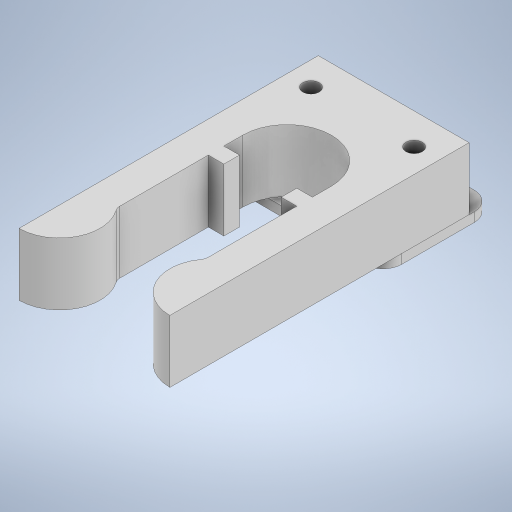
# Autodesk Inventor part: Clip brazo
Saved by Autodesk Inventor 2023 (Build 270158000, 158)
## iProperties
Created: 2022-05-26
Part Number: Clip brazo
Material: Generic
Document SubType Name: Modeling
Designer: juanp
Density: 1 g/cm^3
Appearance: Default
Author: juanp
Autodesk Inventor part; units mm, degrees
ref_plane "YZ Plane" through (0, 0, 0) normal (1, 0, 0) x (0, 1, 0)
ref_plane "XZ Plane" through (0, 0, 0) normal (0, 1, 0) x (-1, 0, 0)
ref_plane "XY Plane" through (0, 0, 0) normal (0, 0, 1) x (1, 0, 0)
sketch "Sketch1" plane through (0, 0, 0) normal (0, 1, 0) x (-1, 0, 0)
  line L0 (14.2, 73.7) -> (-14.2, 73.7) construction
  line L1 (-14.2, 73.7) -> (-14.2, 20)
  line L2 (-14.2, 20) -> (14.2, 20) construction
  line L3 (14.2, 20) -> (14.2, 73.7)
  line L4 (-24.2, 96.0274) -> (-24.2, 20)
  line L5 (24.2, 96.0274) -> (24.2, 20)
  line L6 (-24.2, 20) -> (-14.2, 20)
  line L7 (24.2, 20) -> (14.2, 20)
  line L8 (-24.2, 0) -> (24.2, 0)
  line L9 (24.2, 0) -> (24.2, 20)
  line L10 (24.2, 20) -> (-24.2, 20)
  line L11 (-24.2, 20) -> (-24.2, 0)
  arc A0 (-13.6375, 75.4489) -> (-14.2, 73.7) centre (-11.2, 73.7) ccw
  arc A1 (14.2, 73.7) -> (13.6375, 75.4489) centre (11.2, 73.7) ccw
  arc A2 (24.2, 96.0274) -> (13.6375, 75.4489) centre (24.2, 83.0274) ccw
  arc A3 (-13.6375, 75.4489) -> (-24.2, 96.0274) centre (-24.2, 83.0274) ccw
  line L12 (11.2, 89.334) -> (11.2, 76.7208) construction
  line L13 (-11.2, 89.334) -> (-11.2, 76.7208) construction
  line L14 (-14.2, 73.7) -> (14.2, 73.7)
  line L15 (14.2, 73.7) -> (14.2, 45.3)
  line L16 (14.2, 45.3) -> (-14.2, 45.3)
  line L17 (-14.2, 45.3) -> (-14.2, 73.7)
  line L18 (-14.2, 45.3) -> (-9.2, 45.3)
  line L19 (-9.2, 45.3) -> (-9.2, 40.3)
  line L20 (-9.2, 40.3) -> (-14.2, 40.3)
  line L21 (-14.2, 40.3) -> (-14.2, 45.3)
  line L22 (14.2, 45.3) -> (9.2, 45.3)
  line L23 (9.2, 45.3) -> (9.2, 40.3)
  line L24 (9.2, 40.3) -> (14.2, 40.3)
  line L25 (14.2, 40.3) -> (14.2, 45.3)
  point P0 (0, 0)
  point P1 (0, 0)
  point P2 (-11.2, 83.0274)
  point P3 (11.2, 83.0274)
  point P4 (-11.7, 45.3)
  point P5 (-11.7, 40.3)
  dimension "d0" = 28.4
  dimension "d2" = 3
  dimension "d4" = 3
  dimension "d5" = 3
  dimension "d6" = 20
  dimension "d7" = 10
  dimension "d13" = 53.7
  dimension "d40" = 5
  dimension "d41" = 5
  constraints: 52 end point, 16 equal length, 10 point on circle, 6 horizontal, 6 tangent, 5 midpoint, 5 perpendicular, 4 centre point, 4 vertical, 2 equal radius, 1 coincident, 1 line through centre, 1 point on line, 1 other
  measures "d0" distance of L0.start L0.end
  measures "d2" radius of A0
  measures "d4" distance between parallel lines of L12 L3
  measures "d5" distance between parallel lines of L1 L13
  measures "d6" distance between parallel lines of L8 L10
  measures "d7" distance between parallel lines of L4 L1
  measures "d13" distance of L0.end L1.end
  measures "d40" distance of L23.end L24.end
  measures "d41" distance of point (-11.7, 45.3) point (-11.7, 40.3)
extrude "Extrusion1" add sketch "Sketch1" along normal blind 20 contours L1 L6 L4 A3 A0 | L16 L19 L20 L1 | A1 A2 L5 L7 L3 | L3 L24 L23 L16 | L10 L7 L9 L8 L11 L6
sketch "Sketch2" plane through (0, 20, 0) normal (0, 1, 0) x (1, 0, 0)
  line L0 (-14.2, -20) -> (14.2, -20) projected
  line L1 (0, -20) -> (0, 0) construction
  line L2 (24.2, -96.0274) -> (24.2, 0) projected
  line L3 (-24.2, 0) -> (-24.2, -96.0274) projected
  circle A0 centre (-16.55, -10) radius 2.65
  circle A1 centre (16.55, -10) radius 2.65
  line L4 (0, -10) -> (-24.2, -10) construction
  line L5 (-24.2, 0) -> (-24.2, -96.0274) projected
  line L6 (0, -10) -> (24.2, -10) construction
  dimension "d10" = 5.3
  dimension "d28" = 5
  dimension "d29" = 5
  constraints: 6 end point, 5 point on line, 2 centre point, 2 midpoint, 1 equal radius, 1 perpendicular, 1 vertical
  measures "d10" diameter of A1
  measures "d28" distance edge to line of A0 L3
  measures "d29" distance edge to line of A1 L2
extrude "Extrusion2" cut sketch "Sketch2" against normal through all
fillet "Fillet1" radius 14.2 2 edges at (-14.2, 10, 20) (14.2, 10, 20)
sketch "Sketch4" plane through (0, 0, 0) normal (0, 1, 0) x (1, 0, 0)
  line L0 (-16.55, 0) -> (-16.55, -20) construction
  line L1 (-19.2, 0) -> (-19.2, -20)
  line L2 (-13.9, -20) -> (-13.9, 0)
  arc A0 (-13.9, 0) -> (-19.2, 0) centre (-16.55, 0) ccw
  arc A1 (-19.2, -20) -> (-13.9, -20) centre (-16.55, -20) ccw
  line L3 (16.55, 0) -> (16.55, -20) construction
  line L4 (13.9, 0) -> (13.9, -20)
  line L5 (19.2, -20) -> (19.2, 0)
  arc A2 (19.2, 0) -> (13.9, 0) centre (16.55, 0) ccw
  arc A3 (13.9, -20) -> (19.2, -20) centre (16.55, -20) ccw
  circle A4 centre (-16.55, -10) radius 2.65 projected
  circle A5 centre (16.55, -10) radius 2.65 projected
  circle A6 centre (16.55, -10) radius 2.65 projected
  circle A7 centre (-16.55, -10) radius 2.65 projected
  line L6 (-14.2, -73.7) -> (-14.2, -45.3) projected
  arc A8 (14.2, -34.2) -> (-14.2, -34.2) centre (0, -34.2) ccw projected
  line L7 (14.2, -34.2) -> (14.2, -40.3) projected
  arc A9 (13.6375, -75.4489) -> (14.2, -73.7) centre (11.2, -73.7) ccw projected
  arc A10 (13.6375, -75.4489) -> (24.2, -96.0274) centre (24.2, -83.0274) ccw projected
  line L8 (24.2, -96.0274) -> (24.2, 0) projected
  line L9 (24.2, 0) -> (-24.2, 0) projected
  line L10 (-24.2, 0) -> (-24.2, -96.0274) projected
  arc A11 (-24.2, -96.0274) -> (-13.6375, -75.4489) centre (-24.2, -83.0274) ccw projected
  arc A12 (-14.2, -73.7) -> (-13.6375, -75.4489) centre (-11.2, -73.7) ccw projected
  line L11 (-24.2, -27.65) -> (24.2, -27.65)
  line L12 (24.2, -27.65) -> (24.2, 7.65)
  line L13 (24.2, 7.65) -> (-24.2, 7.65)
  line L14 (-24.2, 7.65) -> (-24.2, -27.65)
  line L15 (-14.2, -45.3) -> (-9.2, -45.3) projected
  line L16 (-9.2, -45.3) -> (-9.2, -40.3) projected
  line L17 (-9.2, -40.3) -> (-14.2, -40.3) projected
  line L18 (-14.2, -40.3) -> (-14.2, -34.2) projected
  line L19 (14.2, -40.3) -> (9.2, -40.3) projected
  line L20 (9.2, -40.3) -> (9.2, -45.3) projected
  line L21 (9.2, -45.3) -> (14.2, -45.3) projected
  line L22 (14.2, -45.3) -> (14.2, -73.7) projected
  point P0 (0, 0)
  point P1 (-16.55, 2.65)
  point P2 (-16.55, -22.65)
  point P3 (-24.2, 0)
  dimension "d15" = 20
  dimension "d16" = 5
  dimension "d17" = 5
  constraints: 24 end point, 10 point on circle, 8 tangent, 6 parallel, 4 centre point, 2 coincident, 2 equal radius, 2 midpoint, 2 point on line, 1 horizontal, 1 perpendicular, 1 vertical
  measures "d15" distance of L0.start L0.end
  measures "d16" distance from line of point (-16.55, 2.65) L13
  measures "d17" distance from line of point (-16.55, -22.65) L11
extrude "Extrusion3" add sketch "Sketch4" against normal blind 3 separate body contours L9 L14 L13 L12 A2 A0 | L1 A1 L2 L9 L4 A3 L5 L8 L11 A8 L10 | A8 L11
sketch "Sketch5" plane through (0, -3, 0) normal (0, -1, 0) x (1, 0, 0)
  line L0 (24.2, 27.65) -> (-24.2, 27.65) projected
  line L1 (0, 27.65) -> (0, -7.65)
  line L2 (-24.2, -7.65) -> (24.2, -7.65) projected
  line L3 (-3, 27.65) -> (-6, 27.65)
  line L4 (-6, 27.65) -> (-6, 18.05)
  line L5 (-6, 18.05) -> (-3, 18.05)
  line L6 (-3, 18.05) -> (-3, 27.65)
  point P0 (0, 0)
  point P1 (-4.5, 27.65)
  point P2 (-4.5, 18.05)
  point P3 (-6, 27.65)
  dimension "d20" = 3
  dimension "d21" = 3
  dimension "d37" = 9.6
  constraints: 10 end point, 4 midpoint, 2 parallel, 1 horizontal, 1 perpendicular, 1 point on line
  measures "d20" distance between parallel lines of L6 L1
  measures "d21" distance between parallel lines of L4 L6
  measures "d37" distance between parallel lines of L0 L5
extrude "Extrusion4" add sketch "Sketch5" along normal blind 20 bodies 2
chamfer "Chamfer1" distance 20 angle 45 1 edges at (-4.5, -3, 18.05)
fillet "Fillet2" radius 6 4 edges at (24.2, -1.5, 27.65) (24.2, -1.5, -7.65) (-24.2, -1.5, 27.65) (-24.2, -1.5, -7.65)
sketch "Sketch6" plane through (-3, -3, 27.65) normal (1, 0, 0) x (0, 0, -1)
  circle A0 centre (7.5, -15) radius 1
  circle A1 centre (7.5, -5) radius 1
  line L0 (7.5, -15) -> (7.5, -5) construction
  line L1 (0, 0) -> (0, -20) projected
  line L2 (6, 0) -> (0, 0) projected
  point P0 (27.65, 3)
  point P1 (0, -10)
  dimension "d33" = 10
  dimension "d34" = 2
  dimension "d38" = 7.5
  dimension "d39" = 5
  constraints: 2 centre point, 2 end point, 1 equal radius, 1 midpoint, 1 vertical
  measures "d33" distance of L0.end L0.start
  measures "d34" diameter of A1
  measures "d38" distance from line of point (0, -10) L0
  measures "d39" distance from line of L0.end L2
extrude "Extrusion5" cut sketch "Sketch6" against normal blind 20 bodies 2
body "Solid1"
body "Solid2"
